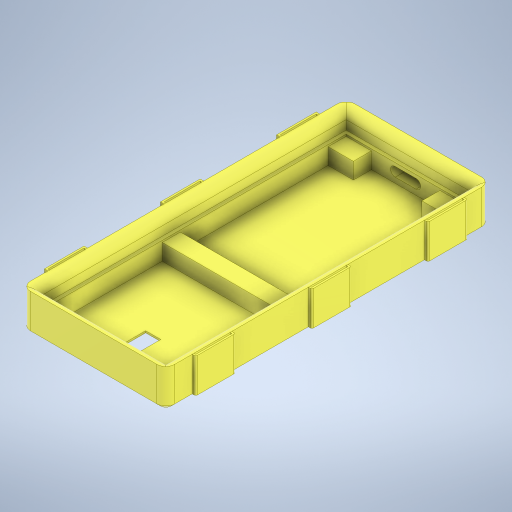
# Autodesk Inventor part: hodinky4
Saved by Autodesk Inventor 2023.2 (Build 272271000, 271)
## iProperties
Created: 2024-01-21
Part Number: hodinky4
Material: Generic
Document SubType Name: Modeling
Designer: marek
Density: 1 g/cm^3
Appearance: Smooth - Yellow
Author: marek
Autodesk Inventor part; units mm, degrees
ref_plane "YZ Plane" through (0, 0, 0) normal (1, 0, 0) x (0, 1, 0)
ref_plane "XZ Plane" through (0, 0, 0) normal (0, 1, 0) x (-1, 0, 0)
ref_plane "XY Plane" through (0, 0, 0) normal (0, 0, 1) x (1, 0, 0)
sketch "Sketch1" plane through (0, 0, 0) normal (0, 1, 0) x (-1, 0, 0)
  line L0 (20, 45) -> (-20, 45)
  line L1 (-20, 45) -> (-20, -45)
  line L2 (-20, -45) -> (20, -45)
  line L3 (20, -45) -> (20, 45)
  line L4 (0, -63) -> (0, 63) projected
  line L5 (-28, 0) -> (28, 0) projected
  point P0 (0, 0)
  dimension "d0" = 40
  dimension "d1" = 90
  constraints: 8 end point, 2 parallel, 1 horizontal, 1 perpendicular, 2 other
  measures "d0" distance of L2.end L1.end
  measures "d1" distance of L1.end L0.end
extrude "Extrusion1" add sketch "Sketch1" along normal blind 0.5
sketch "Sketch2" plane through (0, 0.5, 0) normal (0, 1, 0) x (1, 0, 0)
  line L0 (-20, 45) -> (-20, -45) projected
  line L1 (20, -45) -> (20, 45) projected
  line L2 (-20, -45) -> (20, -45)
  line L3 (20, -45) -> (20, 45)
  line L4 (20, 45) -> (-20, 45)
  line L5 (-20, 45) -> (-20, -45)
  line L6 (-17.5, -42.5) -> (17.5, -42.5)
  line L7 (17.5, -42.5) -> (17.5, 42.5)
  line L8 (17.5, 42.5) -> (-17.5, 42.5)
  line L9 (-17.5, 42.5) -> (-17.5, -42.5)
  point P0 (0, 0)
  dimension "d4" = 2.5
  dimension "d5" = 2.5
  dimension "d6" = 2.5
  dimension "d7" = 2.5
  constraints: 16 end point, 4 parallel, 2 horizontal, 2 perpendicular
  measures "d4" distance between parallel lines of L0 L9
  measures "d5" distance between parallel lines of L1 L7
  measures "d6" distance between parallel lines of L2 L6
  measures "d7" distance between parallel lines of L4 L8
extrude "Extrusion2" add sketch "Sketch2" along normal blind 10
fillet "Fillet2" radius 2.5 4 edges at (-17.5, 10.5, 0) (0, 10.5, -42.5) (17.5, 10.5, 0) (0, 10.5, 42.5)
fillet "Fillet3" radius 2.5 4 edges at (20, 5.25, 45) (-20, 5.25, 45) (20, 5.25, -45) (-20, 5.25, -45)
chamfer "Chamfer8" distance 1 angle 45 8 edges at (0, 0, 45) (19.2678, 0, 44.2678) (20, 0, 0) (19.2678, 0, -44.2678) (0, 0, -45) (-19.2678, 0, -44.2678) (-20, 0, 0) (-19.2678, 0, 44.2678)
sketch "Sketch6" plane through (0, 0.5, 0) normal (0, 1, 0) x (1, 0, 0)
  line L0 (17.5, 42.5) -> (-17.5, 42.5) projected
  line L1 (17.5, -42.5) -> (17.5, 42.5) projected
  line L2 (-17.5, 42.5) -> (17.5, 42.5)
  line L3 (17.5, 42.5) -> (17.5, -42.5)
  line L4 (17.5, -42.5) -> (-17.5, -42.5)
  line L5 (-17.5, -42.5) -> (-17.5, 42.5)
  line L6 (-16.5, -41.5) -> (16.5, -41.5)
  line L7 (16.5, -41.5) -> (16.5, 41.5)
  line L8 (16.5, 41.5) -> (-16.5, 41.5)
  line L9 (-16.5, 41.5) -> (-16.5, -41.5)
  point P0 (0, 0)
  dimension "d39" = 1
  constraints: 16 end point, 4 parallel, 2 perpendicular, 1 horizontal, 3 other
  measures "d39" distance between parallel lines of L4 L6
extrude "Extrusion3" add sketch "Sketch6" along normal blind 5
sketch "Sketch8" plane through (-16.5, 0.5, -41.5) normal (0, 0, 1) x (1, 0, 0)
  line L0 (13.615, 2.785) -> (19.385, 2.785) construction
  line L1 (13.615, 1.5) -> (19.385, 1.5)
  line L2 (19.385, 4.07) -> (13.615, 4.07)
  arc A0 (13.615, 4.07) -> (13.615, 1.5) centre (13.615, 2.785) ccw
  arc A1 (19.385, 1.5) -> (19.385, 4.07) centre (19.385, 2.785) ccw
  line L3 (0, 0) -> (0, 5) projected
  line L4 (33, 0) -> (33, 5) projected
  line L5 (16.5, 18.1) -> (16.5, -3.6) projected
  line L6 (0, 5) -> (33, 5) projected
  line L7 (33, 0) -> (0, 0) projected
  point P0 (16.5, -0.5)
  point P1 (16.5, 2.785)
  point P2 (20.67, 2.785)
  point P3 (12.33, 2.785)
  dimension "d46" = 2.57
  dimension "d50" = 8.34
  dimension "d101" = 1.5
  constraints: 8 end point, 6 point on circle, 4 tangent, 2 centre point, 1 horizontal, 1 midpoint, 1 parallel, 1 other
  measures "d46" distance between parallel lines of L1 L2
  measures "d50" distance of point (20.67, 2.785) point (12.33, 2.785)
  measures "d101" distance between parallel lines of L7 L1
extrude "USB" cut sketch "Sketch8" against normal up to surface (3.5 mm away) contours A0 L2 L5 L1 | L5 L2 A1 L1
sketch "Sketch9" plane through (0, 0.5, 0) normal (0, 1, 0) x (1, 0, 0)
  line L0 (0, 63) -> (0, -63) projected
  line L1 (28, 0) -> (-28, 0) projected
  line L2 (2.1, -34.7) -> (-2.1, -34.7)
  line L3 (-2.1, -34.7) -> (-2.1, -28.5)
  line L4 (-2.1, -28.5) -> (2.1, -28.5)
  line L5 (2.1, -28.5) -> (2.1, -34.7)
  circle A0 centre (-4.5, -32.6) radius 1.5
  circle A1 centre (4.5, -32.6) radius 1.5
  line L6 (16.5, -41.5) -> (-16.5, -41.5) projected
  point P0 (0, 0)
  dimension "d52" = 6.2
  dimension "d53" = 3
  dimension "d54" = 3
  dimension "d57" = 12
  dimension "d58" = 2.4
  dimension "d59" = 2.4
  dimension "d94" = 6.8
  dimension "d95" = 8.9
  dimension "d96" = 8.9
  constraints: 8 end point, 2 centre point, 2 parallel, 1 horizontal, 1 perpendicular, 1 other
  measures "d52" distance of L2.end L3.end
  measures "d53" diameter of A0
  measures "d54" diameter of A1
  measures "d58" distance from line of L5 A1.centre
  measures "d59" distance from line of A0.centre L3
  measures "d94" distance between parallel lines of L6 L2
  measures "d95" distance from line of L6 A0.centre
  measures "d96" distance from line of L6 A1.centre
extrude "MAX30102" cut sketch "Sketch9" against normal up to surface (0.5 mm away) contours L4 L5 L2 L0 | L0 L2 L3 L4
sketch "Sketch10" plane through (20, 10.5, 42.5) normal (1, 0, 0) x (0, 0, -1)
  line L0 (0, 0) -> (85, 0) projected
  line L1 (85, -9.5) -> (0, -9.5) projected
  line L2 (4.8, 0) -> (15.8, 0)
  line L3 (15.8, 0) -> (15.8, -9.5)
  line L4 (15.8, -9.5) -> (4.8, -9.5)
  line L5 (4.8, -9.5) -> (4.8, 0)
  line L6 (0, -9.5) -> (0, 0) projected
  line L7 (37, 10) -> (48, 10)
  line L8 (48, 10) -> (48, -9.5)
  line L9 (48, -9.5) -> (37, -9.5)
  line L10 (37, -9.5) -> (37, 10)
  line L11 (69.2, 10) -> (80.2, 10)
  line L12 (80.2, 10) -> (80.2, -9.5)
  line L13 (80.2, -9.5) -> (69.2, -9.5)
  line L14 (69.2, -9.5) -> (69.2, 10)
  line L15 (85, 0) -> (85, -9.5) projected
  line L16 (-2.5, 0) -> (-2.5, -9.5) projected
  line L17 (87.5, -9.5) -> (87.5, 0) projected
  point P0 (42.5, -10.5)
  point P1 (4.8, -9.5)
  point P2 (74.4653, -20.601)
  point P3 (69.2, 0)
  point P4 (80.2, 0)
  point P5 (37, 0)
  point P6 (48, 0)
  dimension "d66" = 11
  dimension "d76" = 11
  dimension "d77" = 19.5
  dimension "d79" = 11
  dimension "d80" = 19.5
  dimension "d83" = 21.2
  dimension "d84" = 21.2
  dimension "d91" = 7.3
  dimension "d92" = 7.3
  constraints: 24 end point, 6 parallel, 4 point on line, 3 horizontal, 3 perpendicular
  measures "d66" distance of L3.end L4.end
  measures "d76" distance of L8.end L9.end
  measures "d77" distance of L9.end L7.start
  measures "d79" distance of L12.end L13.end
  measures "d80" distance of L13.end L11.start
  measures "d83" distance between parallel lines of L3 L10
  measures "d84" distance between parallel lines of L14 L8
  measures "d91" distance between parallel lines of L16 L5
  measures "d92" distance between parallel lines of L17 L12
extrude "Extrusion6" add sketch "Sketch10" along normal blind 1 contours L0 L3 L1 L5 | L0 L8 L1 L10 | L0 L12 L1 L14
sketch "Sketch11" plane through (20, 10.5, 37.7) normal (0, 1, 0) x (1, 0, 0)
  line L0 (0, 0) -> (0, 11) projected
  line L1 (0, 0.5) -> (0.5, 0.5)
  line L2 (0.5, 0.5) -> (0.5, 10.5)
  line L3 (0.5, 10.5) -> (0, 10.5)
  line L4 (0, 10.5) -> (0, 0.5)
  line L5 (0, 0) -> (1, 0) projected
  line L6 (1, 11) -> (1, 0) projected
  line L7 (0, 11) -> (1, 11) projected
  line L8 (0, 43.2) -> (0, 32.2) projected
  line L9 (0, 32.7) -> (0.5, 32.7)
  line L10 (0.5, 32.7) -> (0.5, 42.7)
  line L11 (0.5, 42.7) -> (0, 42.7)
  line L12 (0, 42.7) -> (0, 32.7)
  line L13 (0, 32.2) -> (1, 32.2) projected
  line L14 (1, 43.2) -> (1, 32.2) projected
  line L15 (0, 43.2) -> (1, 43.2) projected
  line L16 (0, 75.4) -> (0, 64.4) projected
  line L17 (0, 64.9) -> (0.5, 64.9)
  line L18 (0.5, 64.9) -> (0.5, 74.9)
  line L19 (0.5, 74.9) -> (0, 74.9)
  line L20 (0, 74.9) -> (0, 64.9)
  line L21 (1, 75.4) -> (1, 64.4) projected
  line L22 (0, 64.4) -> (1, 64.4) projected
  line L23 (0, 75.4) -> (1, 75.4) projected
  point P0 (-20, 37.7)
  point P1 (0, 10.5)
  point P2 (0, 74.9)
  point P3 (0, 42.7)
  dimension "d70" = 0.5
  dimension "d71" = 0.5
  dimension "d72" = 0.5
  dimension "d85" = 0.5
  dimension "d86" = 0.5
  dimension "d87" = 0.5
  dimension "d88" = 0.5
  dimension "d89" = 0.5
  dimension "d90" = 0.5
  constraints: 24 end point, 6 parallel, 3 horizontal, 3 perpendicular, 3 point on line
  measures "d70" distance between parallel lines of L5 L1
  measures "d71" distance between parallel lines of L6 L2
  measures "d72" distance between parallel lines of L7 L3
  measures "d85" distance between parallel lines of L13 L9
  measures "d86" distance between parallel lines of L14 L10
  measures "d87" distance between parallel lines of L15 L11
  measures "d88" distance between parallel lines of L21 L18
  measures "d89" distance between parallel lines of L22 L17
  measures "d90" distance between parallel lines of L23 L19
extrude "Extrusion7" cut sketch "Sketch11" against normal up to surface (9.5 mm away) contours L0 L3 L2 L1 | L11 L10 L9 L8 | L19 L18 L17 L16
fillet "Fillet4" radius 0.5 6 edges at (21, 5.75, 37.7) (21, 5.75, 26.7) (21, 5.75, 5.5) (21, 5.75, -5.5) (21, 5.75, -26.7) (21, 5.75, -37.7)
mirror "Mirror1" about plane through (0, 0, 0) normal (1, 0, 0) of "Extrusion6", "Extrusion7"
sketch "Sketch13" plane through (0, 0.5, 0) normal (0, 1, 0) x (1, 0, 0)
  line L0 (-16.5, -41.5) -> (-16.5, 41.5) projected
  line L1 (-16.5, 41.5) -> (-9.5, 41.5)
  line L2 (-9.5, 41.5) -> (-9.5, 36.5)
  line L3 (-9.5, 36.5) -> (-16.5, 36.5)
  line L4 (-16.5, 36.5) -> (-16.5, 41.5)
  line L5 (16.5, 41.5) -> (16.5, -41.5) projected
  line L6 (16.5, 41.5) -> (9.5, 41.5)
  line L7 (9.5, 41.5) -> (9.5, 36.5)
  line L8 (9.5, 36.5) -> (16.5, 36.5)
  line L9 (16.5, 36.5) -> (16.5, 41.5)
  line L10 (-16.5, -9.5) -> (16.5, -9.5)
  line L11 (16.5, -9.5) -> (16.5, -4.5)
  line L12 (16.5, -4.5) -> (-16.5, -4.5)
  line L13 (-16.5, -4.5) -> (-16.5, -9.5)
  line L14 (-16.5, 41.5) -> (16.5, 41.5) projected
  line L15 (0, 63.0032) -> (0, -63.0032) projected
  line L16 (29.4, 0) -> (-29.4, 0) projected
  point P0 (0, 0)
  point P1 (-16.5, -4.5)
  point P2 (16.5, -9.5)
  dimension "d103" = 5
  dimension "d105" = 5
  dimension "d106" = 5
  dimension "d110" = 51
  dimension "d111" = 19
  constraints: 24 end point, 6 parallel, 3 horizontal, 3 perpendicular, 2 point on line, 1 other
  measures "d103" distance of L1.end L2.end
  measures "d105" distance of L7.end L6.end
  measures "d106" distance of L11.end L10.end
  measures "d110" distance between parallel lines of L14 L10
  measures "d111" distance between parallel lines of L7 L2
extrude "Extrusion9" add sketch "Sketch13" along normal blind 4.5 contours L0 L12 L15 L10 | L15 L12 L5 L10 | L0 L1 L2 L3 | L6 L5 L8 L7
body "Solid1"
